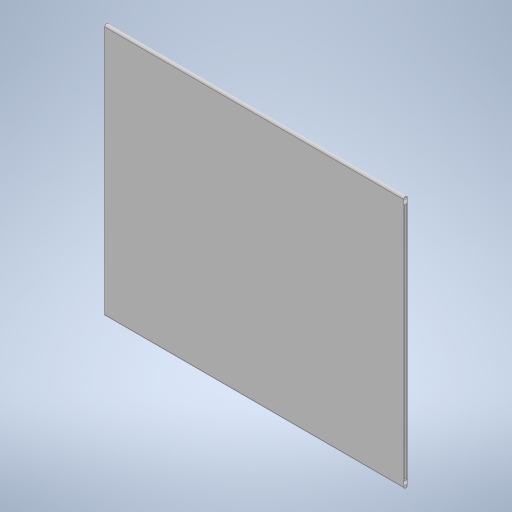
# Autodesk Inventor part: Conveyer Belt
Saved by Autodesk Inventor 2024 (Build 280153000, 153)
## iProperties
Created: 2024-09-16
Part Number: Conveyer Belt
Material: Generic
Document SubType Name: Modeling
Designer: srira
Density: 1 g/cm^3
Appearance: Default
Author: srira
Autodesk Inventor part; units mm, degrees
ref_plane "YZ Plane" through (0, 0, 0) normal (1, 0, 0) x (0, 1, 0)
ref_plane "XZ Plane" through (0, 0, 0) normal (0, 1, 0) x (-1, 0, 0)
ref_plane "XY Plane" through (0, 0, 0) normal (0, 0, 1) x (1, 0, 0)
sketch "Sketch1" plane through (0, 0, 0) normal (1, 0, 0) x (0, 1, 0)
  circle A0 centre (500, 0) radius 5
  circle A1 centre (-500, 0) radius 5
  arc A2 (500, -7.5) -> (500, 7.5) centre (500, 0) ccw
  arc A3 (-500, 7.5) -> (-500, -7.5) centre (-500, 0) ccw
  line L0 (500, -7.5) -> (-500, -7.5)
  line L1 (500, 7.5) -> (-500, 7.5)
  line L2 (-480, 5) -> (480, 5)
  line L3 (480, 5) -> (480, -5)
  line L4 (480, -5) -> (-480, -5)
  line L5 (-480, -5) -> (-480, 5)
  line L6 (-480, 5) -> (480, -5) construction
  line L7 (480, 5) -> (-480, -5) construction
  point P0 (0, 0)
  dimension "d0" = 10
  dimension "d1" = 10
  dimension "d2" = 15
  dimension "d3" = 15
  dimension "d4" = 1000
  dimension "d5" = 1000
  dimension "d6" = 960
  dimension "d7" = 10
  constraints: 16 end point, 4 centre point, 4 point on circle, 2 coincident, 2 midpoint, 2 parallel, 1 horizontal, 1 perpendicular
  measures "d0" diameter of A0
  measures "d1" diameter of A1
  measures "d2" diameter of A2
  measures "d3" diameter of A3
  measures "d4" distance of L0.start L0.end
  measures "d5" distance of L1.start L1.end
  measures "d6" distance of L3.end L4.end
  measures "d7" distance of L2.end L3.end
extrude "Extrusion1" add sketch "Sketch1" along normal blind 1200
body "Solid1"
